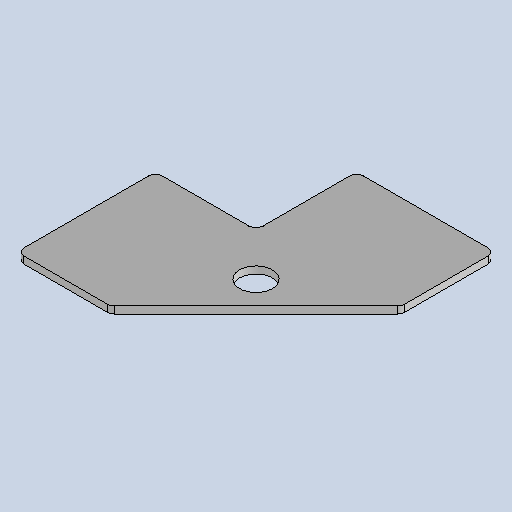
# Autodesk Inventor part: GNH 081 leg support
Saved by Autodesk Inventor 2025.1 (Build 291241020, 241B)
## iProperties
Created: 2025-03-06
Part Number: GNH 081 leg support
Material: Stainless Steel
Document SubType Name: Sheet Metal
Designer: user
Density: 8 g/cm^3
Flat Pattern Width: 6.89203 cm
Flat Pattern Length: 14.2083 cm
Flat Pattern Area: 97.9242 cm^2
Sheet Metal Rule: AISI304 3mm Die 32
Sheet Metal Width: 68.920 mm
Sheet Metal Length: 142.083 mm
Sheet Metal Area: 9792.422 mm^2
Appearance: Default
Author: user
Autodesk Inventor part; units mm, degrees
ref_plane "YZ Plane" through (0, 0, 0) normal (1, 0, 0) x (0, 1, 0)
ref_plane "XZ Plane" through (0, 0, 0) normal (0, 1, 0) x (-1, 0, 0)
ref_plane "XY Plane" through (0, 0, 0) normal (0, 0, 1) x (1, 0, 0)
sketch "Sketch2" plane through (0, 0, 0) normal (0, 0, 1) x (1, 0, 0)
  line L0 (0, 0) -> (40, 0) construction
  line L1 (40, 0) -> (40, -40) construction
  line L2 (40, -40) -> (0, -40) construction
  line L3 (0, -40) -> (0, 0) construction
  line L4 (43, 0) -> (43, -43)
  line L5 (43, -43) -> (0, -43)
  line L6 (0, -43) -> (0, -102.2254)
  line L7 (0, -102.2254) -> (40, -102.2254)
  line L8 (40, -102.2254) -> (102.2254, -40)
  line L9 (102.2254, -40) -> (102.2254, 0)
  line L10 (102.2254, 0) -> (43, 0)
  line L11 (43, -43) -> (71.1127, -71.1127) construction
  circle A0 centre (61.2132, -61.2132) radius 7
  dimension "d7" = 40
  dimension "d8" = 40
  dimension "d9" = 3
  dimension "d10" = 3
  dimension "d11" = 14
  dimension "d12" = 30
  dimension "d13" = 14
  measures "d7" distance of L1.end L2.end
  measures "d8" distance of L0.end L1.end
  measures "d9" distance between parallel lines of L5 L2
  measures "d10" distance between parallel lines of L1 L4
  measures "d11" diameter of A0
  measures "d12" distance of A0.centre L1.end
  measures "d13" distance from line of A0.centre L8
extrude "Plate2" add sketch "Sketch2" along normal blind 3
fillet "Corner Round3" radius 3 7 edges at (0, -102.2254, 1.5) (0, -43, 1.5) (43, -43, 1.5) (43, 0, 1.5) (102.2254, 0, 1.5) (102.2254, -40, 1.5) (40, -102.2254, 1.5)
feature "Corner Round4" [suppressed]
sketch "Sketch3" plane through (43, -103.468, 3) normal (-0.7071068, 0.7071068, 0) x (-0.7071068, -0.7071068, 0)
  line L0 (-85.5147, 0) -> (0, 0)
  line L1 (0, 0) -> (0, -20)
  line L2 (0, -20) -> (-85.5147, -20)
  line L3 (-85.5147, -20) -> (-85.5147, 0)
  constraints: 8 end point
equation "\"d8\" = d7"
equation "\"d10\" = d9"
equation "\"d13\" = d11"
equation "\"d14\" = Thickness"
equation "\"BendReliefWidth\" = Thickness"
equation "\"BendReliefDepth\" = 0.5 * Thickness"
equation "\"CornerReliefSize\" = 4 * Thickness"
equation "\"MinimumRemnant\" = 2 * Thickness"
equation "\"TransitionRadius\" = BendRadius"
equation "\"JacobiRadiusSize\" = BendRadius"
equation "\"GapSize\" = Thickness"
equation "\"Thickness\" = 3"
equation "\"BendRadius\" = 5"
body "Solid2"
